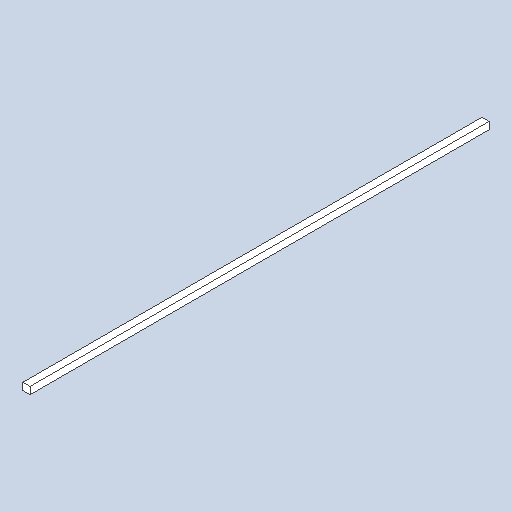
# Autodesk Inventor part: stock
Saved by Autodesk Inventor 2023 (Build 270158000, 158)
## iProperties
Created: 2019-08-08
Part Number: stock
Material: Generic
Document SubType Name: Modeling
Designer: shenglab2
Density: 1 g/cm^3
Appearance: Default
Author: shenglab2
Autodesk Inventor part; units mm, degrees
ref_plane "YZ Plane" through (0, 0, 0) normal (1, 0, 0) x (0, 1, 0)
ref_plane "XZ Plane" through (0, 0, 0) normal (0, 1, 0) x (-1, 0, 0)
ref_plane "XY Plane" through (0, 0, 0) normal (0, 0, 1) x (1, 0, 0)
sketch "Sketch1" plane through (0, 0, 0) normal (0, 0, 1) x (1, 0, 0)
  line L0 (2.3813, -2.3813) -> (-2.3813, -2.3813)
  line L1 (-2.3813, -2.3813) -> (-2.3813, 2.3812)
  line L2 (-2.3813, 2.3812) -> (2.3813, 2.3813)
  line L3 (2.3813, 2.3813) -> (2.3813, -2.3813)
  line L4 (2.3813, -2.3813) -> (-2.3813, 2.3812) construction
  line L5 (-2.3813, -2.3813) -> (2.3813, 2.3813) construction
  point P0 (0, 0)
  dimension "d0" = 4.7625
  dimension "d1" = 4.7625
  constraints: 12 end point, 2 midpoint, 2 parallel, 1 horizontal, 1 perpendicular
  measures "d0" distance of L1.end L2.end
  measures "d1" distance of L0.end L1.end
extrude "Extrusion1" add sketch "Sketch1" along normal blind 304.8
equation "\"d1\" = d0"
body "Solid1"
